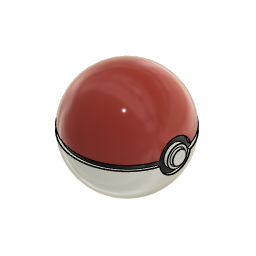
Pokeball 3D exercice (Autodesk Fusion 360 design; units mm, degrees)
Autodesk Fusion 360 part; units mm, degrees
note: some values were not read from the file. Set by a fixed rule: which sketch regions a step uses; which face or edge a step refers to.
sketch "Esquisse1" plane through (0, 0, 0) normal (0, 0, 1) x (1, 0, 0)
  circle A0 centre (6, -6) radius 5
  line L0 (12.2202, -6) -> (0, -6)
  line L1 (0, -6) -> (-0.5, -6)
  line L2 (5.7277, -14.6619) -> (5.7277, 2.6619)
  line L3 (5.7277, 2.6619) -> (6.2723, 2.6619)
  line L4 (6.2723, 2.6619) -> (6.2723, -14.6619)
  line L5 (6.2723, -14.6619) -> (5.7277, -14.6619)
  line L6 (5.7277, -14.6619) -> (6.2723, 2.6619) construction
  line L7 (5.7277, 2.6619) -> (6.2723, -14.6619) construction
  point P0 (6, -6)
  dimension "d1" = 10
  constraint coincident origin A0.centre
  constraint parallel L0 L1
  constraint perpendicular L2 L3
  constraint parallel L2 L4
  constraint parallel L3 L5
  constraint coincident L6 P0
  constraint coincident L7 P0
  constraint coincident P0 A0.centre
  measures "d1" diameter of A0
sketch "Esquisse2" plane through (0, 0, 0) normal (0, 0, 1) x (1, 0, 0)
sketch "Esquisse3" plane through (0, 0, 0) normal (1, 0, 0) x (0, 1, 0)
  circle A0 centre (0, 0) radius 5
  line L0 (0, 0) -> (0, 6.5)
  line L1 (0, 6.5) -> (0, -6.5)
  line L2 (9.0773, 0.2342) -> (-9.0773, 0.2342)
  line L3 (-9.0773, 0.2342) -> (-9.0773, -0.2342)
  line L4 (-9.0773, -0.2342) -> (9.0773, -0.2342)
  line L5 (9.0773, -0.2342) -> (9.0773, 0.2342)
  line L6 (9.0773, 0.2342) -> (-9.0773, -0.2342) construction
  line L7 (-9.0773, 0.2342) -> (9.0773, -0.2342) construction
  dimension "d5" = 10
  constraint coincident A0.centre L0.start
  constraint vertical L0
  constraint parallel L0 L1
  constraint horizontal L2
  constraint perpendicular L2 L3
  constraint parallel L2 L4
  constraint parallel L3 L5
  constraint coincident L6 A0.centre
  constraint coincident L7 A0.centre
  measures "d5" diameter of A0
revolve "Révolution2" add sketch "Esquisse3" angle 360 about axis through (0, 0, 6.5) along (0, 0, -1) contours A0 L0 L1 L2 | A0 L1 L4 picked at (3.3029, 0.4634) picked at (3.3029, -0.4634) makes body 1 at (-4.2649, 2.4623, 0.8649) makes body 2 at (-4.2649, -2.4623, -0.8649)
shell "Coque2" thickness 0.25 removed faces 2 at (1.3016, 1.038, 0.2342) at (0.2723, 0.634, -0.2342) on bodies 1 2
sketch "Esquisse4" plane through (0, 0, 0) normal (0, 1, 0) x (1, 0, 0)
sketch "Esquisse5" plane through (0, 0, 0) normal (1, 0, 0) x (0, 1, 0)
  circle A0 centre (0, 0) radius 4.75
  line L0 (0, 6.5) -> (0, -6.1788)
  line L1 (-4.743, 0.2576) -> (4.743, 0.2576)
  dimension "d8" = 9.5
  constraint coincident A0.centre origin
  constraint vertical L0
  constraint coincident A0 L1.start
  constraint coincident A0 L1.end
  constraint horizontal L1
  measures "d8" diameter of A0
revolve "Révolution3" add sketch "Esquisse5" angle 360 about axis through (0, 0, 6.5) along (0, 0, -1) separate body contours A0 L0 L1 | A0 L0 L1 picked at (0.2253, -3.0647) picked at (3.1352, 0.4741) makes body 3
ref_plane "Plan de construction2" through (5, 0, 0) normal (1, 0, 0) x (0, 1, 0)
sketch "Esquisse6" plane through (5, 0, 0) normal (1, 0, 0) x (0, 1, 0)
  circle A0 centre (0, 0) radius 1.5
  circle A1 centre (0, 0) radius 1
  circle A2 centre (0, 0) radius 0.75
  circle A3 centre (0, 0) radius 0.675
  dimension "d12" = 3
  dimension "d13" = 2
  dimension "d14" = 1.5
  dimension "d15" = 1.35
  constraint coincident A0.centre A1.centre
  constraint concentric A0 A1
  constraint concentric A1 A3
  measures "d12" diameter of A0
  measures "d13" diameter of A1
  measures "d14" diameter of A2
  measures "d15" diameter of A3
extrude "Extrusion1" cut sketch "Esquisse6" along normal up to surface contours A0 | A1 | A2 | A3 end surface at (-4.0784, -2.3547, -0.62) on bodies 3 bodies 1 2
extrude "Extrusion2" add sketch "Esquisse6" along normal up to surface separate body contours A1 end surface at (-4.0784, -2.3547, -0.62) on bodies 3 makes body 4
extrude "Extrusion3" add sketch "Esquisse6" along normal blind 0.2 and the other way up to surface separate body contours A3 second end surface at (-4.0784, -2.3547, -0.62) on bodies 3 makes body 5
fillet "Congé1" radius 0.025 6 edges at (-4.9945, 0, 0.2342) (4.7697, 0, 1.5) (-4.9945, 0, -0.2342) (4.7697, 0, -1.5) (5, -0.9323, -0.3616) (5.2, -0.6293, -0.2441) on bodies 1 2 4 5
